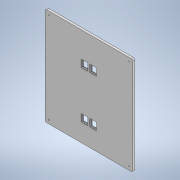
# Autodesk Inventor part: Etage 1
Saved by Autodesk Inventor 2020.1 (Build 241239000, 239)
## iProperties
Created: 2019-11-15
Part Number: Etage 1
Material: Generic
Document SubType Name: Modeling
Designer: Admin
Density: 1 g/cm^3
Appearance: Default
Author: Admin
Autodesk Inventor part; units mm, degrees
ref_plane "YZ Plane" through (0, 0, 0) normal (1, 0, 0) x (0, 1, 0)
ref_plane "XZ Plane" through (0, 0, 0) normal (0, 1, 0) x (-1, 0, 0)
ref_plane "XY Plane" through (0, 0, 0) normal (0, 0, 1) x (1, 0, 0)
sketch "Sketch1" plane through (0, 0, 0) normal (0, 0, 1) x (1, 0, 0)
  line L0 (-118.6456, 73.2494) -> (122.9544, 73.2494)
  line L1 (122.9544, 73.2494) -> (122.9544, -196.7506)
  line L2 (122.9544, -196.7506) -> (-118.6456, -196.7506)
  line L3 (-118.6456, -196.7506) -> (-118.6456, 73.2494)
  circle A0 centre (-108.6456, 63.2494) radius 1.5
  circle A1 centre (112.9544, 63.2494) radius 1.5
  circle A2 centre (-108.6456, -186.7506) radius 1.5
  circle A3 centre (112.9544, -186.7506) radius 1.5
  point P0 (0, 0)
  dimension "d0" = 241.6
  dimension "d1" = 270
  dimension "d2" = 10
  dimension "d3" = 10
  dimension "d4" = 3
  dimension "d5" = 10
  dimension "d6" = 10
  dimension "d7" = 3
  dimension "d8" = 10
  dimension "d9" = 10
  dimension "d10" = 3
  dimension "d11" = 10
  dimension "d12" = 10
  dimension "d13" = 3
  constraints: 8 end point, 4 centre point, 2 parallel, 1 horizontal, 1 perpendicular
  measures "d0" distance of L0.start L0.end
  measures "d1" distance of L0.end L1.end
  measures "d2" distance from line of L0 A0.centre
  measures "d3" distance from line of L3 A0.centre
  measures "d4" diameter of A0
  measures "d5" distance from line of L0 A1.centre
  measures "d6" distance from line of L1 A1.centre
  measures "d7" diameter of A1
  measures "d8" distance from line of L1 A3.centre
  measures "d9" distance from line of L2 A3.centre
  measures "d10" diameter of A3
  measures "d11" distance from line of L3 A2.centre
  measures "d12" distance from line of L2 A2.centre
  measures "d13" diameter of A2
extrude "Extrusion1" add sketch "Sketch1" along normal blind 6
fillet "Fillet1" radius 4 4 edges at (-118.6456, 73.2494, 3) (122.9544, 73.2494, 3) (122.9544, -196.7506, 3) (-118.6456, -196.7506, 3)
sketch "Sketch2" plane through (0, 0, 0) normal (0, 0, -1) x (-1, 0, 0)
  line L0 (-22.9544, 3.2494) -> (-4.9544, 3.2494)
  line L1 (-4.9544, 3.2494) -> (-4.9544, -16.7506)
  line L2 (-4.9544, -16.7506) -> (-22.9544, -16.7506)
  line L3 (-22.9544, -16.7506) -> (-22.9544, 3.2494)
  line L4 (18.6456, -16.7506) -> (0.6456, -16.7506)
  line L5 (0.6456, -16.7506) -> (0.6456, 3.2494)
  line L6 (0.6456, 3.2494) -> (18.6456, 3.2494)
  line L7 (18.6456, 3.2494) -> (18.6456, -16.7506)
  line L8 (-22.9544, -146.7506) -> (-4.9544, -146.7506)
  line L9 (-4.9544, -146.7506) -> (-4.9544, -126.7506)
  line L10 (-4.9544, -126.7506) -> (-22.9544, -126.7506)
  line L11 (-22.9544, -126.7506) -> (-22.9544, -146.7506)
  line L12 (0.6456, -126.7506) -> (18.6456, -126.7506)
  line L13 (18.6456, -126.7506) -> (18.6456, -146.7506)
  line L14 (18.6456, -146.7506) -> (0.6456, -146.7506)
  line L15 (0.6456, -146.7506) -> (0.6456, -126.7506)
  line L16 (-122.9544, -192.7506) -> (-122.9544, 69.2494) projected
  line L17 (-118.9544, 73.2494) -> (114.6456, 73.2494) projected
  line L18 (118.6456, 69.2494) -> (118.6456, -192.7506) projected
  line L19 (114.6456, -196.7506) -> (-118.9544, -196.7506) projected
  point P0 (0, 0)
  dimension "d17" = 100
  dimension "d18" = 18
  dimension "d19" = 20
  dimension "d20" = 70
  dimension "d21" = 18
  dimension "d22" = 100
  dimension "d23" = 20
  dimension "d24" = 70
  dimension "d25" = 70
  dimension "d26" = 70
  dimension "d27" = 100
  dimension "d28" = 100
  dimension "d29" = 20
  dimension "d30" = 18
  dimension "d31" = 20
  constraints: 32 end point, 8 parallel, 4 horizontal, 4 perpendicular, 1 point on line
  measures "d17" distance between parallel lines of L16 L3
  measures "d18" distance of L1.end L2.end
  measures "d19" distance of L2.end L0.start
  measures "d20" distance between parallel lines of L17 L0
  measures "d21" distance of L5.end L6.end
  measures "d22" distance between parallel lines of L18 L7
  measures "d23" distance of L6.end L4.start
  measures "d24" distance from line of L17 L6.end
  measures "d25" distance between parallel lines of L19 L10
  measures "d26" distance between parallel lines of L19 L12
  measures "d27" distance between parallel lines of L16 L11
  measures "d28" distance between parallel lines of L18 L13
  measures "d29" distance of L10.end L8.start
  measures "d30" distance of L12.start L12.end
  measures "d31" distance of L14.end L12.start
extrude "Extrusion3" cut sketch "Sketch2" against normal blind 6
body "Solid1"
